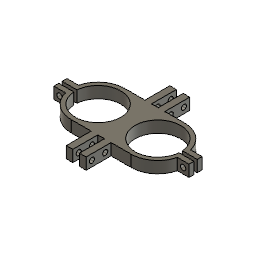
Flywheel Base (Autodesk Fusion 360 design; units mm, degrees)
part number: 2026-08-23-00-31-53-753
Autodesk Fusion 360 part; units mm, degrees
sketch "Sketch1" plane through (0, 0, 0) normal (0, 1, 0) x (1, 0, 0)
  line L0 (1.75, 0) -> (22.5, 0)
  arc A0 (-33.6984, -4) -> (-33.6984, 4) centre (-18, 0) ccw
  arc A1 (-31.6635, -1) -> (-31.6635, 1) centre (-18, 0) ccw
  line L1 (-33.6984, 4) -> (-40.6984, 4)
  line L2 (-40.6984, 4) -> (-40.6984, 1)
  line L3 (-40.6984, 1) -> (-31.6635, 1)
  line L4 (-33.6984, -4) -> (-40.6984, -4)
  line L5 (-40.6984, -4) -> (-40.6984, -1)
  line L6 (-40.6984, -1) -> (-31.6635, -1)
  line L7 (-18, 0) -> (-40.6984, 0) construction
  circle A2 centre (-18, 0) radius 12.9205 construction
  line L8 (0, -16.2) -> (0, 16.2)
  line L9 (0, 16.2) -> (-18, 16.2)
  line L10 (0, -16.2) -> (-18, -16.2)
  line L11 (0, 16.2) -> (18, 16.2)
  line L12 (33.6984, -4) -> (40.6984, -4)
  arc A3 (31.6635, 1) -> (31.6635, -1) centre (18, 0) ccw
  circle A4 centre (18, 0) radius 12.9205 construction
  line L13 (40.6984, -4) -> (40.6984, -1)
  line L14 (40.6984, -1) -> (31.6635, -1)
  line L15 (40.6984, 4) -> (40.6984, 1)
  line L16 (18, 0) -> (40.6984, 0) construction
  line L17 (40.6984, 1) -> (31.6635, 1)
  line L18 (0, -16.2) -> (18, -16.2)
  line L19 (33.6984, 4) -> (40.6984, 4)
  line L20 (0, -16.2) -> (0, 16.2)
  arc A5 (33.6984, 4) -> (33.6984, -4) centre (18, 0) ccw
  point P0 (-1.75, 0)
  dimension "d2" = 18
  dimension "d16" = 7
  dimension "d17" = 3
  dimension "d18" = 7
  dimension "d19" = 3
  dimension "d20" = 25.841
  dimension "d21" = 32.4
  dimension "d22" = 13.7
  dimension "d23" = 16.2
  constraint coincident A0.centre A1.centre
  constraint horizontal L1
  constraint perpendicular L1 L2
  constraint perpendicular L2 L3
  constraint parallel L3 L4
  constraint perpendicular L4 L5
  constraint parallel L3 L7
  constraint concentric A0 A2
  constraint midpoint L8 origin
  constraint vertical L8
  constraint coincident A0 L9.end
  constraint tangent A0 L9
  constraint perpendicular L8 L9
  constraint coincident A0 L10.end
  constraint tangent A0 L10
  constraint symmetric A0.start L8 L12.start
  constraint symmetric A0.end L8 L19.start
  constraint symmetric L0.start L8 P0
  constraint symmetric A1.start L8 A3.end
  constraint symmetric A1.end L8 A3.start
  constraint symmetric A0 L8 A5
  constraint symmetric A1 L8 A3
  constraint symmetric L1.end L8 L15.start
  constraint symmetric L2.end L8 L15.end
  constraint symmetric L4.end L8 L12.end
  constraint symmetric L5.end L8 L13.end
  constraint symmetric A0.centre L8 A3.centre
  constraint symmetric L7.end L8 L16.end
  constraint symmetric A2 L8 A4
  constraint symmetric L10.start L8 L18.start
  constraint symmetric L9.start L8 L11.start
  constraint symmetric L8 L9.end L11.end
  constraint symmetric L8 L10.end L18.end
  measures "d2" distance of origin A0.centre
  measures "d16" distance of A0.end L1.end
  measures "d17" distance of L1.end L2.end
  measures "d18" distance of A0.start L4.end
  measures "d19" distance of L4.end L5.end
  measures "d20" diameter of A2
  measures "d21" distance of L8.start L8.end
  measures "d22" radius of A1
  measures "d23" radius of A0
extrude "Extrude1" add sketch "Sketch1" along normal blind 7
hole "Hole1" at (-37.1984, 3.5, -4) direction (0, 0, 1) diameter 3.2 depth 8 tip angle 180
hole "Hole2" at (37.1984, 3.5, 4) direction (0, 0, -1) diameter 3.2 depth 8 tip angle 180
sketch "Sketch3" plane through (0, 0, 16.2) normal (0, 0, 1) x (1, 0, 0)
  line L0 (-18, 0) -> (18, 0)
  line L1 (18, 0) -> (18, 7)
  line L2 (18, 7) -> (-18, 7)
  line L3 (-18, 7) -> (-18, 0)
  line L4 (0, 0) -> (0, 7) construction
  line L5 (-2, 7) -> (-6, 7)
  line L6 (-6, 7) -> (-6, 0)
  line L7 (-6, 0) -> (-2, 0)
  line L8 (-2, 0) -> (-2, 7)
  line L9 (2, 7) -> (6, 7)
  line L10 (6, 7) -> (6, 0)
  line L11 (6, 0) -> (2, 0)
  line L12 (2, 0) -> (2, 7)
  dimension "d35" = 4
  dimension "d36" = 7
  dimension "d37" = 2
  dimension "d38" = 4
  dimension "d39" = 7
  dimension "d40" = 2
  constraint coincident L4.start origin
  constraint midpoint L2 L4.end
  constraint horizontal L5
  constraint vertical L6
  constraint horizontal L7
  constraint vertical L8
  constraint coincident L2 L5.start
  constraint horizontal L9
  constraint vertical L10
  constraint horizontal L11
  constraint vertical L12
  constraint coincident L2 L9.start
  measures "d35" distance of L5.start L5.end
  measures "d36" distance of L5.start L7.end
  measures "d37" distance of L4 L8
  measures "d38" distance of L9.start L9.end
  measures "d39" distance of L9.start L11.end
  measures "d40" distance of L4 L12
sketch "Sketch4" plane through (0, 0, -16.2) normal (0, 0, -1) x (-1, 0, 0)
  line L0 (-18, 0) -> (18, 0)
  line L1 (18, 0) -> (18, 7)
  line L2 (18, 7) -> (-18, 7)
  line L3 (-18, 7) -> (-18, 0)
  line L4 (0, 0) -> (0, 7) construction
  line L5 (-6, 7) -> (-2, 7)
  line L6 (-2, 7) -> (-2, 0)
  line L7 (-2, 0) -> (-6, 0)
  line L8 (-6, 0) -> (-6, 7)
  line L9 (2, 7) -> (6, 7)
  line L10 (6, 7) -> (6, 0)
  line L11 (6, 0) -> (2, 0)
  line L12 (2, 0) -> (2, 7)
  dimension "d41" = 2
  dimension "d42" = 2
  dimension "d43" = 4
  dimension "d44" = 4
  constraint coincident L4.start origin
  constraint midpoint L2 L4.end
  constraint horizontal L5
  constraint vertical L6
  constraint horizontal L7
  constraint vertical L8
  constraint coincident L0 L6.end
  constraint coincident L2 L5.start
  constraint horizontal L9
  constraint vertical L10
  constraint horizontal L11
  constraint vertical L12
  constraint coincident L0 L10.end
  constraint coincident L2 L9.start
  measures "d41" distance of L4 L6
  measures "d42" distance of L4 L12
  measures "d43" distance of L5.start L5.end
  measures "d44" distance of L9.start L9.end
extrude "Extrude2" add sketch "Sketch4" along normal blind 15 contours L0 L2 L5 L6 L7 L8 | L0 L2 L9 L10 L11 L12
extrude "Extrude3" add sketch "Sketch3" along normal blind 15 contours L0 L2 L5 L6 L7 L8 | L0 L2 L9 L10 L11 L12
hole "Hole3" at (-6, 3.5, -27.7) direction (1, 0, 0) diameter 3.1 depth 12 tip angle 180
hole "Hole4" at (-6, 3.5, -19.7) direction (1, 0, 0) diameter 3.1 depth 12 tip angle 180
hole "Hole5" at (6, 3.5, 27.7) direction (-1, 0, 0) diameter 3.1 depth 12 tip angle 180
hole "Hole6" at (6, 3.5, 19.7) direction (-1, 0, 0) diameter 3.1 depth 12 tip angle 180
